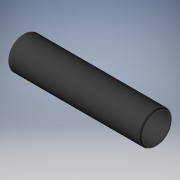
# Autodesk Inventor part: 04R-3.25550SR
Saved by Autodesk Inventor 2019 (Build 230136000, 136)
## iProperties
Created: 2023-01-12
Part Number: 04R-3.25550SR
Material: Generic
Catalog Web Link: www.cadenas.de
Description: Tube-Original Line - Standard Air Cylinders
Vendor: BIMBA
Document SubType Name: Modeling
Designer: psAdmin
Manufacturer: BIMBA
Mass: 3.10566 g
Surface Area: 106.126 cm^2
Volume: 3.10566 cm^3
Density: 1 g/cm^3
Appearance: PSOLRGB-180-180-180
Category: PARTsolutions
Company: BIMBA
Title: 04R-3.25550SR
Author: Cadenas PARTsolutions
Comments: Original Line - Standard Air Cylinders
PSOL_IDENT_0: {$CADENAS_DATA/23d-libs/bimba/bimba_brand/bimba_imperial/bimba_full_line/original_line_cylinders/sta
PSOL_IDENT_1: ndard_air_cylinders/tube.prj},205 {VTYP=3D},{NB=04R-3.25550SR},{LINA=04R-3.25550SR},{NN=Tube},{DATE=
PSOL_IDENT_2: 23.12.2022 11:35:28},{GEOMDATE=12.07.2022 08:39:00},{VERSION=},{LINEID=40},{WBVAR=MNT,ACTING,NR,L,FO
PSOL_IDENT_3: URHOLES,SR,K},{WBNUMERIC=L,FOURHOLES}  {NB=04R-3.25550SR},{LINA=04R-3.25550SR},{KT=DUMMY},{PN=04R-3.
PSOL_IDENT_4: 25550SR},{BORE=0.75000000},{BOREPN=04},{MNT=},{MNTALG='' , 'Front Nose' , 'BF' , 'Front Block' , 'BF
PSOL_IDENT_5: T' , 'Front Trunnion' , 'A' , 'Adjustable Stroke'},{ACTING=R},{ACTINGALG= '' , 'Single Acting' , 'R'
PSOL_IDENT_6: , 'Reverse/Double Acting' },{NR=},{NRALG= '' , 'N/A' },{L=3.2555},{OD=0.8075},{ODN=0.8050},{ODP=0.8
PSOL_IDENT_7: 625},{ODB=0.8325},{ID=0.7615},{DV=0.00000000},{LV=0.00000000},{LV1=0.00000000},{G=0.0300},{FOURHOLES=
PSOL_IDENT_8: 0},{AA=0.3750},{BB=0.0940},{SR=SR},{SRALG= 'C' , 'Carbon Steel Rod' , 'SR' , '303 Stainless Steel Ro
PSOL_IDENT_9: d' , '' , '303 Stainless Steel Rod'},{KALG= '', 'Standard' , 'K' , 'Ports Rotated 90deg' },{K=}
NB: 04R-3.25550SR
NN: Tube
NT: Original Line - Standard Air Cylinders
NBSYN: $PN.
LINA: 04R-3.25550SR
CATALOG: Bimba Products
BORE: 0
BOREPN: 04
MNT: Front Nose
MNTALG: '' , 'Front Nose' , 'BF' , 'Front Block' , 'BFT' , 'Front Trunnion' , 'A' , 'Adjustable Stroke'
ACTING: Reverse/Double Acting
NR: N/A
L: 3.2555
ODN: 0.805
ODP: 0.8625
ODB: 0.8325
ID: 0.7615
DV: 0
LV: 0
LV1: 0
G: 0.03
FOURHOLES: 0
AA: 0.375
BB: 0.094
SR: 303 Stainless Steel Rod
K: Standard
SUPPLIER: BIMBA
ARTICLENO: 04R-3.25550SR
BOMINFO: 04R-3.25550SR
CREATOR: CADENAS GmbH
Autodesk Inventor part; units mm, degrees
sketch "Sketch_1" plane through (0, 0, 0) normal (0, 0, 1) x (1, 0, 0)
  line L0 (82.6897, 0) -> (0, 0)
  arc A0 (-0.6395, 9.3472) -> (-0.6395, 9.1676) centre (-0.5497, 9.2574) ccw
  line L1 (-0.6395, 9.1676) -> (-0.381, 8.9091)
  line L2 (-0.381, 8.9091) -> (0, 8.9091)
  line L3 (0, 8.9091) -> (0.762, 9.671)
  line L4 (0.762, 9.671) -> (81.9277, 9.671)
  line L5 (81.9277, 9.671) -> (82.6897, 8.9091)
  line L6 (82.6897, 8.9091) -> (83.0707, 8.9091)
  line L7 (83.0707, 8.9091) -> (83.3292, 9.1676)
  arc A1 (83.3292, 9.1676) -> (83.3292, 9.3472) centre (83.2394, 9.2574) ccw
  line L8 (83.3292, 9.3472) -> (82.6443, 10.0321)
  arc A2 (82.6443, 10.0321) -> (82.1055, 10.2553) centre (82.1055, 9.4933) ccw
  line L9 (82.1055, 10.2553) -> (0.5842, 10.2553)
  arc A3 (0.5842, 10.2553) -> (0.0454, 10.0321) centre (0.5842, 9.4933) ccw
  line L10 (0.0454, 10.0321) -> (-0.6395, 9.3472)
  constraints: 22 end point, 8 point on circle, 4 centre point
revolve "Revolution1" add sketch "Sketch_1" angle 360 about axis through (82.6897, 0, 0) along (1, 0, 0)
ref_plane "cp1_XY" through (41.3448, 0, 10.2553) normal (1, 0, 0) x (0, 0, -1)
ref_plane "cp1_YZ" through (41.3448, 0, 10.2553) normal (0, 0, -1) x (0, 1, 0)
ref_plane "cp1_ZX" through (41.3448, 0, 10.2553) normal (0, 1, 0) x (1, 0, 0)
ref_plane "cp2_XY" through (41.3448, 10.2553, 0) normal (1, 0, 0) x (0, 0, -1)
ref_plane "cp2_YZ" through (41.3448, 10.2553, 0) normal (0, 0, -1) x (0, 1, 0)
ref_plane "cp2_ZX" through (41.3448, 10.2553, 0) normal (0, 1, 0) x (1, 0, 0)
ref_plane "cp3_XY" through (41.3448, 0, -10.2553) normal (1, 0, 0) x (0, 0, -1)
ref_plane "cp3_YZ" through (41.3448, 0, -10.2553) normal (0, 0, -1) x (0, 1, 0)
ref_plane "cp3_ZX" through (41.3448, 0, -10.2553) normal (0, 1, 0) x (1, 0, 0)
ref_plane "cp4_XY" through (41.3448, -10.2553, 0) normal (1, 0, 0) x (0, 0, -1)
ref_plane "cp4_YZ" through (41.3448, -10.2553, 0) normal (0, 0, -1) x (0, 1, 0)
ref_plane "cp4_ZX" through (41.3448, -10.2553, 0) normal (0, 1, 0) x (1, 0, 0)
ref_plane "tube_front_XY" through (0, 0, 0) normal (1, 0, 0) x (0, 0, -1)
ref_plane "tube_front_YZ" through (0, 0, 0) normal (0, 0, -1) x (0, 1, 0)
ref_plane "tube_front_ZX" through (0, 0, 0) normal (0, 1, 0) x (1, 0, 0)
ref_plane "tube_rear_XY" through (82.6897, 0, 0) normal (1, 0, 0) x (0, 0, -1)
ref_plane "tube_rear_YZ" through (82.6897, 0, 0) normal (0, 0, -1) x (0, 1, 0)
ref_plane "tube_rear_ZX" through (82.6897, 0, 0) normal (0, 1, 0) x (1, 0, 0)
body "Solid1"
